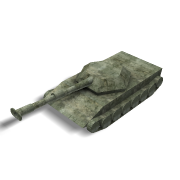
# Autodesk Inventor part: Simple Tank 1
Saved by Autodesk Inventor 2019 (Build 230136000, 136)
## iProperties
Created: 2022-03-19
Part Number: Simple Tank 1
Material: Generic
Document SubType Name: Modeling
Designer: DuyKhanh
Density: 1 g/cm^3
Appearance: Precast Smooth
Author: DuyKhanh
Autodesk Inventor part; units mm, degrees
note: some values were not read from the file. Chosen so that the rebuilt part matches the saved one: side of "Thicken1".
ref_plane "YZ Plane" through (0, 0, 0) normal (1, 0, 0) x (0, 1, 0)
ref_plane "XZ Plane" through (0, 0, 0) normal (0, 1, 0) x (-1, 0, 0)
sketch "Sketch1" plane through (0, 0, 0) normal (1, 0, 0) x (0, 1, 0)
  circle A0 centre (354.253, -253.3243) radius 350
  circle A1 centre (556.3839, 580.1777) radius 300
  point P0 (0, 0)
  dimension "d0" = 700
  dimension "d6" = 600
  constraints: 2 centre point
  measures "d0" diameter of A0
  measures "d6" diameter of A1
extrude "Extrusion1" add sketch "Sketch1" along normal blind 250 contours A0
pattern_linear "Rectangular Pattern1" count 6 spacing 750 along (0, 0, -1) of "Extrusion1"
extrude "Extrusion2" add sketch "Sketch1" along normal blind 250 contours A1
pattern_linear "Rectangular Pattern2" count 2 spacing 5300 along (0, 0, -1) of "Extrusion2"
sketch "Sketch2" plane through (250, 354.253, -253.3243) normal (1, 0, 0) x (0, 0, -1)
  circle A0 centre (-833.502, 202.1309) radius 300 construction
  circle A1 centre (0, 0) radius 350 construction
  circle A2 centre (3750, 0) radius 350 construction
  circle A3 centre (4466.498, 202.1309) radius 300 construction
  line L0 (-779.9159, 497.3063) -> (31.5119, 350)
  circle A4 centre (0, 0) radius 350 projected
  line L1 (31.5119, 350) -> (3713.5123, 350)
  circle A5 centre (3750, 0) radius 350 projected
  line L2 (3713.5123, 350) -> (4404.6202, 495.6801)
  circle A6 centre (4466.498, 202.1309) radius 300 projected
  line L3 (4567.1596, -80.4771) -> (3867.4385, -329.7093)
  line L4 (3750, -350) -> (0, -350)
  line L5 (-102.1762, -334.7537) -> (-921.0816, -84.8008)
  arc A7 (4567.1596, -80.4771) -> (4404.6202, 495.6801) centre (4466.498, 202.1309) ccw
  arc A8 (3750, -350) -> (3867.4385, -329.7093) centre (3750, 0) ccw
  arc A9 (-102.1762, -334.7537) -> (0, -350) centre (0, 0) ccw
  arc A10 (-779.9159, 497.3063) -> (-921.0816, -84.8008) centre (-833.502, 202.1309) ccw
  point P0 (-253.3243, -354.253)
  constraints: 18 tangent, 16 point on circle, 12 end point, 4 centre point, 2 concentric
surface extrude "ExtrusionSrf1" sketch "Sketch2" against normal blind 250 shown no curves L1 L2 A7 L3 A8 L4 A9 L5 A10 L0
thicken "Thicken1" operation new thickness 15 both sides no extend neighbours no toward (0, 1, 0) faces at (166.6667, 704.253, -1512.1697) (83.3333, 802.4572, 256.1157) (166.6667, 347.4583, 795.4683) (83.3333, 102.817, 121.8203) (83.3333, 4.3597, -244.6847) (166.6667, 4.253, -2753.3243) (83.3333, 4.3441, -4011.3077) (166.6667, 190.6986, -4587.2435) (166.6667, 823.917, -4855.5649) (166.6667, 752.8131, -4197.2059)
sketch "Sketch3" plane through (0, 556.3839, 580.1777) normal (-1, 0, 0) x (0, 0, 1)
  line L0 (-811.71, -261.8835) -> (566.1285, 143.1504)
  line L1 (566.1285, 143.1504) -> (-811.71, 638.5937)
  line L2 (-811.71, 638.5937) -> (-5757.1093, 638.5937)
  line L3 (-5757.1093, 638.5937) -> (-5660.6198, 35.0438)
  line L4 (-5660.6198, 35.0438) -> (-4738.5152, -261.8835)
  line L5 (-4738.5152, -261.8835) -> (-811.71, -261.8835)
  point P0 (-580.1777, -556.3839)
  constraints: 12 end point, 1 horizontal, 1 parallel
extrude "Extrusion3" add sketch "Sketch3" along normal blind 1500 separate body
mirror "Mirror1" about plane through (-1500, 759.5511, -2117.6331) normal (-1, 0, 0) bodies 3 1 2
sketch "Sketch4" plane through (0, 1194.9776, -231.5323) normal (0, 1, 0) x (1, 0, 0)
  line L0 (-2927.3926, 1657.8575) -> (-2213.6963, 2894.0158)
  line L1 (-2213.6963, 2894.0158) -> (-786.3037, 2894.0158)
  line L2 (-786.3037, 2894.0158) -> (-72.6074, 1657.8575)
  line L3 (-72.6074, 1657.8575) -> (-786.3037, 421.6992)
  line L4 (-786.3037, 421.6992) -> (-2213.6963, 421.6992)
  line L5 (-2213.6963, 421.6992) -> (-2927.3926, 1657.8575)
  line L6 (0, 4945.3993) -> (-3000, 4945.3993) projected
  point P0 (0, -231.5323)
  point P1 (-1500, 1657.8575)
  point P2 (-1500, 2894.0158)
  point P3 (-1500, 4945.3993)
  constraints: 12 end point, 2 midpoint, 1 horizontal, 1 vertical alignment, 13 other
extrude "Extrusion4" add sketch "Sketch4" along normal blind 250 draft 20 bodies 3
sketch "Sketch5" plane through (0, 1444.9776, -231.5323) normal (0, 1, 0) x (1, 0, 0)
  line L0 (-2266.2309, 2985.0083) -> (-733.7691, 2985.0083) projected
  line L1 (-3032.4618, 1657.8575) -> (-2266.2309, 2985.0083) projected
  line L2 (-2266.2309, 330.7066) -> (-3032.4618, 1657.8575) projected
  line L3 (-733.7691, 330.7066) -> (-2266.2309, 330.7066) projected
  line L4 (32.4618, 1657.8575) -> (-733.7691, 330.7066) projected
  line L5 (-733.7691, 2985.0083) -> (32.4618, 1657.8575) projected
  point P0 (0, -231.5323)
extrude "Extrusion5" add sketch "Sketch5" along normal blind 450 draft -45 bodies 3
ref_plane "Work Plane1" through (-786.3037, 1444.9776, -562.239) normal (0, 0.0871557, 0.9961947) x (-1, 0, 0)
sketch "Sketch6" plane through (-786.3037, 1444.9776, -562.239) normal (0, 0.0871557, 0.9961947) x (-1, 0, 0)
  circle A0 centre (713.6963, -217.5077) radius 185
  line L0 (207.273, -487.5077) -> (1220.1196, -487.5077) projected
  point P0 (-786.3037, 1488.4814)
  point P1 (713.6963, -487.5077)
  dimension "d23" = 370
  dimension "d24" = 270
  constraints: 1 centre point, 1 midpoint, 1 vertical alignment
  measures "d23" diameter of A0
  measures "d24" distance from line of A0.centre L0
extrude "Extrusion6" add sketch "Sketch6" along normal blind 800 draft -2 and the other way blind 400 draft 7 bodies 3
sketch "Sketch7" plane through (-1500, 1731.3822, 215.7597) normal (0, 0.0871557, 0.9961947) x (1, 0, 0)
  circle A0 centre (0, 0) radius 142.5
  point P0 (1500, -1705.9891)
  dimension "d29" = 285
  constraints: 1 centre point
  measures "d29" diameter of A0
extrude "Extrusion7" add sketch "Sketch7" along normal blind 800 bodies 3
sketch "Sketch8" plane through (-1500, 1801.1068, 1012.7155) normal (0, 0.0871557, 0.9961947) x (1, 0, 0)
  circle A0 centre (-1.1454, 28.8135) radius 187.5
  point P0 (1500, -1705.9891)
  dimension "d32" = 375
  constraints: 1 centre point
  measures "d32" diameter of A0
extrude "Extrusion8" add sketch "Sketch8" along normal blind 500 bodies 3
sketch "Sketch9" plane through (-1501.1454, 1873.3885, 1508.3016) normal (0, 0.0871557, 0.9961947) x (1, 0, 0)
  circle A0 centre (1.1454, -28.8135) radius 142.5 projected
  point P0 (1501.1454, -1734.8026)
extrude "Extrusion9" add sketch "Sketch9" along normal blind 1200 bodies 3
sketch "Sketch10" plane through (-1500, 1949.2716, 2706.2465) normal (0, 0.0871557, 0.9961947) x (1, 0, 0)
  circle A0 centre (0, 0) radius 175
  point P0 (1500, -1705.9891)
  dimension "d37" = 350
  constraints: 1 centre point
  measures "d37" diameter of A0
extrude "Extrusion10" add sketch "Sketch10" along normal blind 800 bodies 3
sketch "Sketch11" plane through (-1500, 2018.9962, 3503.2022) normal (0, 0.0871557, 0.9961947) x (1, 0, 0)
  line L0 (-215.0292, 0) -> (215.0292, 0) construction
  line L1 (-215.0292, -179.0163) -> (215.0292, -179.0163)
  line L2 (215.0292, 179.0163) -> (-215.0292, 179.0163)
  arc A0 (-215.0292, 179.0163) -> (-215.0292, -179.0163) centre (-215.0292, 0) ccw
  arc A1 (215.0292, -179.0163) -> (215.0292, 179.0163) centre (215.0292, 0) ccw
  circle A2 centre (0, 0) radius 137.5
  point P0 (1500, -1705.9891)
  dimension "d40" = 275
  constraints: 8 end point, 4 point on circle, 4 tangent, 3 centre point, 1 coincident, 1 horizontal, 1 midpoint, 1 parallel
  measures "d40" diameter of A2
extrude "Extrusion11" add sketch "Sketch11" against normal blind 50 bodies 3
extrude "Extrusion12" cut sketch "Sketch11" against normal blind 4535.75 contours A2 bodies 3
body "Solid1"
body "Srf1"
body "Solid2"
body "Solid3"
